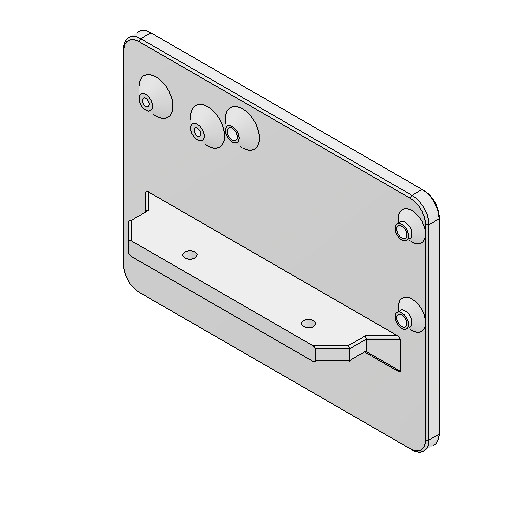
# Autodesk Inventor part: temp-logger-side-plate
Saved by Autodesk Inventor 2026 (Build 300175050, 175E)
## iProperties
Created: 2025-07-16
Part Number: temp-logger-side-plate
Material: ABS Plastic
Document SubType Name: Modeling
Designer: kuzmin
Density: 1.06 g/cm^3
Appearance: Smooth - White
Author: kuzmin
Autodesk Inventor part; units mm, degrees
ref_plane "YZ Plane" through (0, 0, 0) normal (1, 0, 0) x (0, 1, 0)
ref_plane "XZ Plane" through (0, 0, 0) normal (0, 1, 0) x (-1, 0, 0)
ref_plane "XY Plane" through (0, 0, 0) normal (0, 0, 1) x (1, 0, 0)
sketch "Sketch1" plane through (0, 0, 0) normal (0, 0, 1) x (1, 0, 0)
  line L0 (-45, 32.5) -> (45, 32.5)
  line L1 (45, 32.5) -> (45, -32.5)
  line L2 (45, -32.5) -> (-45, -32.5)
  line L3 (-45, -32.5) -> (-45, 32.5)
  line L4 (-38.5, 26.5) -> (38.5, 26.5) construction
  line L5 (38.5, 26.5) -> (38.5, -26.5) construction
  line L6 (38.5, -26.5) -> (-38.5, -26.5) construction
  line L7 (-38.5, -26.5) -> (-38.5, 26.5) construction
  circle A0 centre (-38.5, 26.5) radius 2
  circle A1 centre (38.5, 26.5) radius 2
  circle A2 centre (38.5, -26.5) radius 2
  circle A3 centre (-38.5, -26.5) radius 2
  point P0 (0, 0)
  point P1 (45, 0)
  point P2 (0, 32.5)
  point P3 (38.5, 0)
  point P4 (0, 26.5)
  dimension "d0" = 90
  dimension "d1" = 65
  dimension "d2" = 77
  dimension "d3" = 53
  dimension "d14" = 4
  constraints: 16 end point, 8 coincident, 4 centre point, 4 midpoint, 4 parallel, 3 equal radius, 2 horizontal, 2 horizontal alignment, 2 perpendicular, 2 vertical alignment
  measures "d0" distance of L0.start L0.end
  measures "d1" distance of L0.end L1.end
  measures "d2" distance of L4.start L4.end
  measures "d3" distance of L4.end L5.end
  measures "d14" diameter of A0
extrude "Extrusion1" add sketch "Sketch1" along normal blind 4 contours L0 L1 L2 L3 | A0 | A1 | A2 | A3
fillet "Fillet1" radius 5 4 edges at (45, 32.5, 2) (45, -32.5, 2) (-45, -32.5, 2) (-45, 32.5, 2)
chamfer "Chamfer2" distance 0.5 angle 45 9 edges at (0, 32.5, 0) (-43.5355, 31.0355, 0) (-45, 0, 0) (-43.5355, -31.0355, 0) (0, -32.5, 0) (43.5355, -31.0355, 0) (45, 0, 0) (43.5355, 31.0355, 0) (0, 32.5, 4)
sketch "Sketch2" plane through (0, 0, 0) normal (0, 0, 1) x (1, 0, 0)
  line L0 (40.5, 25.1) -> (40.5, 2.5) construction
  line L1 (45, -27.5) -> (45, 27.5) projected
  line L2 (-40, -32.5) -> (40, -32.5) projected
  circle A0 centre (40.5, 25.1) radius 2
  circle A1 centre (40.5, 2.5) radius 2
  line L3 (40.5, 25.1) -> (-9.5, 25.1) construction
  circle A2 centre (-9.5, 25.1) radius 2
  point P0 (0, 0)
  dimension "d23" = 22.6
  dimension "d24" = 4.5
  dimension "d25" = 35
  dimension "d26" = 4
  dimension "d39" = 50
  constraints: 5 coincident, 4 end point, 3 centre point, 2 equal radius, 1 horizontal, 1 vertical
  measures "d23" distance of L0.start L0.end
  measures "d24" distance between parallel lines of L1 L0
  measures "d25" distance from line of L2 L0.end
  measures "d26" diameter of A0
  measures "d39" distance of L3.start L3.end
extrude "Extrusion3" add sketch "Sketch2" along normal blind 7
hole "Hole2" at (40.5, 25.1, 0) at (40.5, 2.5, 0) at (-9.5, 25.1, 0) direction (0, 0, 1) diameter 3 end through all
chamfer "Chamfer3" distance 3 angle 45 1 edges at (-11.5, 25.1, 4)
chamfer "Chamfer4" distance 2 angle 45 2 edges at (38.5, 25.1, 4) (38.5, 2.5, 4)
sketch "Sketch3" plane through (0, 0, 0) normal (0, 0, -1) x (-1, 0, 0)
  line L0 (19.76, 20.5) -> (35, 20.5) construction
  line L1 (35, 20.5) -> (35, 2.5) construction
  line L2 (35, 2.5) -> (19.76, 2.5) construction
  line L3 (19.76, 2.5) -> (19.76, 20.5) construction
  circle A0 centre (19.76, 20.5) radius 2
  circle A1 centre (35, 20.5) radius 2
  line L4 (40, 32.5) -> (-40, 32.5) projected
  line L5 (45, -27.5) -> (45, 27.5) projected
  point P0 (0, 0)
  dimension "d43" = 15.24
  dimension "d44" = 18
  dimension "d45" = 4
  dimension "d58" = 12
  dimension "d79" = 10
  constraints: 8 end point, 4 coincident, 2 centre point, 2 parallel, 1 equal radius, 1 horizontal, 1 perpendicular
  measures "d43" distance of L0.start L0.end
  measures "d44" distance of L0.end L1.end
  measures "d45" diameter of A0
  measures "d58" distance between parallel lines of L4 L0
  measures "d79" distance from line of L5 point (35, 20.5)
extrude "MAX" add sketch "Sketch3" against normal blind 7
hole "Hole3" at (-19.76, 20.5, 0) at (-35, 20.5, 0) direction (0, 0, 1) diameter 2 end through all
chamfer "Chamfer5" distance 3 angle 45 2 edges at (-33, 20.5, 4) (-17.76, 20.5, 4)
sketch "Sketch4" plane through (0, 0, 4) normal (0, 0, 1) x (1, 0, 0)
  line L0 (-33, -5) -> (32, -5)
  line L1 (32, -5) -> (32, -9)
  line L2 (32, -9) -> (-33, -9)
  line L3 (-33, -9) -> (-33, -5)
  line L4 (40, 32.5) -> (-40, 32.5) projected
  line L5 (-45, 27.5) -> (-45, -27.5) projected
  point P0 (0, 0)
  dimension "d59" = 37.5
  dimension "d60" = 65
  dimension "d61" = 4
  dimension "d62" = 12
  constraints: 8 end point, 2 parallel, 1 horizontal, 1 perpendicular
  measures "d59" distance between parallel lines of L0 L4
  measures "d60" distance of L1.end L2.end
  measures "d61" distance of L2.end L0.start
  measures "d62" distance between parallel lines of L5 L3
extrude "Extrusion5" add sketch "Sketch4" along normal blind 15
sketch "Sketch5" plane through (-33, -5, 4) normal (0, 1, 0) x (1, 0, 0)
  line L0 (-7, 0) -> (73, 0) projected
  line L1 (18, -10) -> (53, -10) construction
  line L2 (-12, 3.5) -> (-12, 0.5) projected
  point P0 (33, 4)
  point P1 (-12, 2)
  dimension "d65" = 30
  dimension "d66" = 10
  dimension "d80" = 65
  constraints: 2 coincident, 2 end point, 1 horizontal, 1 midpoint
  measures "d65" horizontal distance of L2.end point (18, -10)
  measures "d66" distance from line of point (18, -10) L0
  measures "d80" horizontal distance of point (-12, 2) L1.end
hole "Hole4" at (-15, -5, 14) at (20, -5, 14) direction (0, -1, 0) diameter 3 end through all
chamfer "Chamfer6" distance 5 angle 45 5 edges at (-0.5, -9, 4) (32, -7, 4) (-33, -7, 4) (-33, -7, 19) (32, -7, 19)
fillet "Fillet2" radius 0.5 12 edges at (-35.5, -11.5, 6.5) (-33, -9, 11.5) (-30.5, -9, 16.5) (29.5, -9, 16.5) (32, -9, 11.5) (34.5, -11.5, 6.5) (-35.5, -5, 6.5) (34.5, -5, 6.5) (32, -5, 11.5) (29.5, -5, 16.5) (-30.5, -5, 16.5) (-33, -5, 11.5)
equation "\"d0\" = width"
equation "\"d1\" = hight"
equation "\"d4\" = thickness"
equation "\"d27\" = thickness + bump"
equation "\"d46\" = thickness + bump"
equation "\"width\" = 90"
equation "\"hight\" = 65"
equation "\"thickness\" = 4"
equation "\"bump\" = 3"
body "Solid1"
